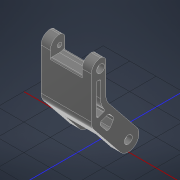
# Autodesk Inventor part: Swing-Arm B
Saved by Autodesk Inventor 2022.2 (Build 262287010, 287A)
## iProperties
Created: 2022-03-22
Part Number: Swing-Arm B
Material: ABS-Kunststoff
Document SubType Name: Modeling
Designer: sleib
Density: 1.06 g/cm^3
Appearance: Glatt - Schwarz
Author: sleib
Autodesk Inventor part; units mm, degrees
ref_plane "YZ Plane" through (0, 0, 0) normal (1, 0, 0) x (0, 1, 0)
ref_plane "XZ Plane" through (0, 0, 0) normal (0, 1, 0) x (-1, 0, 0)
ref_plane "XY Plane" through (0, 0, 0) normal (0, 0, 1) x (1, 0, 0)
sketch "SwingArm B" plane through (0, 0, 0) normal (0, 0, 1) x (1, 0, 0)
  arc A0 (25.4839, 28) -> (19.2029, 25.7813) centre (25.4839, 18) ccw
  arc A1 (37.33, 17) -> (31.049, 14.7813) centre (37.33, 7) ccw
  circle A2 centre (0, 0) radius 8 construction
  arc A3 (-5.0248, 6.2251) -> (5.0248, -6.2251) centre (0, 0) ccw
  line L0 (31.049, 14.7813) -> (5.0248, -6.2251)
  line L1 (19.2029, 25.7813) -> (-5.0248, 6.2251)
  line L2 (57, 28) -> (25.4839, 28)
  line L3 (60, 17) -> (37.33, 17)
  circle A4 centre (57, 21) radius 7 construction
  arc A5 (64, 21) -> (57, 28) centre (57, 21) ccw
  arc A6 (60, 17) -> (64, 21) centre (60, 21) ccw
  circle A7 centre (0, 0) radius 1.7
  circle A8 centre (57, 21) radius 1.7
  line L4 (57, 21) -> (26.0163, 21) construction
  line L5 (26.0163, 21) -> (0, 0) construction
  line L6 (22.6557, 20.0016) -> (24.0687, 16.0016)
  line L7 (23.4391, 13.7792) -> (20.7308, 11.5931)
  line L8 (18.4256, 11.4466) -> (14.8137, 13.6716)
  line L9 (14.6065, 16.9307) -> (19.5137, 20.8917)
  arc A9 (22.6557, 20.0016) -> (19.5137, 20.8917) centre (20.7699, 19.3355) ccw
  arc A10 (23.4391, 13.7792) -> (24.0687, 16.0016) centre (22.1829, 15.3355) ccw
  arc A11 (18.4256, 11.4466) -> (20.7308, 11.5931) centre (19.4746, 13.1494) ccw
  arc A12 (14.6065, 16.9307) -> (14.8137, 13.6716) centre (15.8627, 15.3744) ccw
  line L10 (22.1532, 27.429) -> (27.6033, 12) construction
  line L11 (37.33, 21) -> (60, 21) construction
  arc A13 (60, 21) -> (57, 24) centre (57, 21) ccw construction
  line L12 (57, 24) -> (25.4839, 24) construction
  arc A14 (25.4839, 24) -> (21.7153, 22.6688) centre (25.4839, 18) ccw construction
  line L13 (21.7153, 22.6688) -> (-2.5124, 3.1125) construction
  arc A15 (-2.5124, 3.1125) -> (2.5124, -3.1125) centre (0, 0) ccw construction
  line L14 (2.5124, -3.1125) -> (28.5366, 17.8939) construction
  arc A16 (37.33, 21) -> (28.5366, 17.8939) centre (37.33, 7) ccw construction
  line L15 (49.9641, 21.75) -> (50.2223, 22.75)
  line L16 (27.3731, 18.6564) -> (25.9565, 22.6669)
  line L17 (48.9958, 21) -> (37.33, 21)
  line L18 (49.254, 24) -> (26.8994, 24)
  arc A17 (37.33, 21) -> (28.917, 18.1902) centre (37.33, 7) ccw
  arc A18 (27.3731, 18.6564) -> (28.917, 18.1902) centre (28.316, 18.9895) ccw
  arc A19 (26.8994, 24) -> (25.9565, 22.6669) centre (26.8994, 23) ccw
  arc A20 (50.2223, 22.75) -> (49.254, 24) centre (49.254, 23) ccw
  arc A21 (48.9958, 21) -> (49.9641, 21.75) centre (48.9958, 22) ccw
  line L19 (17.0601, 18.9112) -> (22.0849, 12.6862) construction
  line L20 (13.0503, 15.6745) -> (18.0751, 9.4494) construction
  dimension "d0" = 3.4
  dimension "d1" = 3.4
  dimension "d2" = 57
  dimension "d3" = 21
  dimension "d4" = 141.09
  dimension "d5" = 4
  dimension "d6" = 7
  dimension "d7" = 4
  dimension "d10" = 10
  dimension "d11" = 10
  dimension "d13" = 2
  dimension "d14" = 2
  dimension "d42" = 16
  dimension "d43" = 4
  dimension "d45" = 1
  dimension "d46" = 4
  dimension "d49" = 20
  measures "d0" diameter of A7
  measures "d1" diameter of A8
  measures "d2" horizontal distance of L5.end L4.start
  measures "d3" vertical distance of L5.end L4.start
  measures "d4" angle of L5 L4
  measures "d5" distance from line of L3 L4.start
  measures "d6" distance from line of L4.start L2
  measures "d7" radius of A6
  measures "d10" radius of A1
  measures "d11" radius of A0
  measures "d13" radius of A9
  measures "d14" radius of A10
  measures "d42" diameter of A2
  measures "d43" distance between parallel lines of L3 L11
  measures "d45" radius of A20
  measures "d46" distance between parallel lines of L6 L16
  measures "d49" distance from line of point (0, 0) L20
sketch "Skizze1" plane through (0, 0, 0) normal (1, 0, 0) x (0, 1, 0)
  circle A0 centre (0, 0) radius 18
  arc A1 (52, 21) -> (54, 17) centre (57, 21) ccw
  line L0 (52, 21) -> (52, 28)
  arc A2 (25.4839, 28) -> (19.2029, 25.7813) centre (25.4839, 18) ccw
  arc A3 (37.33, 17) -> (31.049, 14.7813) centre (37.33, 7) ccw
  circle A4 centre (0, 0) radius 8 construction
  arc A5 (-5.0248, 6.2251) -> (5.0248, -6.2251) centre (0, 0) ccw
  line L1 (31.049, 14.7813) -> (5.0248, -6.2251)
  line L2 (19.2029, 25.7813) -> (-5.0248, 6.2251)
  line L3 (57, 28) -> (25.4839, 28)
  line L4 (60, 17) -> (37.33, 17)
  circle A6 centre (57, 21) radius 7 construction
  arc A7 (64, 21) -> (57, 28) centre (57, 21) ccw
  arc A8 (60, 17) -> (64, 21) centre (60, 21) ccw
  circle A9 centre (0, 0) radius 1.7
  circle A10 centre (57, 21) radius 1.7
  line L5 (57, 21) -> (26.0163, 21) construction
  line L6 (26.0163, 21) -> (0, 0) construction
  line L7 (22.6557, 20.0016) -> (24.0687, 16.0016)
  line L8 (23.4391, 13.7792) -> (20.7308, 11.5931)
  line L9 (18.4256, 11.4466) -> (14.8137, 13.6716)
  line L10 (14.6065, 16.9307) -> (19.5137, 20.8917)
  arc A11 (22.6557, 20.0016) -> (19.5137, 20.8917) centre (20.7699, 19.3355) ccw
  arc A12 (23.4391, 13.7792) -> (24.0687, 16.0016) centre (22.1829, 15.3355) ccw
  arc A13 (18.4256, 11.4466) -> (20.7308, 11.5931) centre (19.4746, 13.1494) ccw
  arc A14 (14.6065, 16.9307) -> (14.8137, 13.6716) centre (15.8627, 15.3744) ccw
  line L11 (22.1532, 27.429) -> (27.6033, 12) construction
  line L12 (37.33, 21) -> (60, 21) construction
  arc A15 (60, 21) -> (57, 24) centre (57, 21) ccw construction
  line L13 (57, 24) -> (25.4839, 24) construction
  arc A16 (25.4839, 24) -> (21.7153, 22.6688) centre (25.4839, 18) ccw construction
  line L14 (21.7153, 22.6688) -> (-2.5124, 3.1125) construction
  arc A17 (-2.5124, 3.1125) -> (2.5124, -3.1125) centre (0, 0) ccw construction
  line L15 (2.5124, -3.1125) -> (28.5366, 17.8939) construction
  arc A18 (37.33, 21) -> (28.5366, 17.8939) centre (37.33, 7) ccw construction
  line L16 (49.9641, 21.75) -> (50.2223, 22.75)
  line L17 (27.3731, 18.6564) -> (25.9565, 22.6669)
  line L18 (48.9958, 21) -> (37.33, 21)
  line L19 (49.254, 24) -> (26.8994, 24)
  arc A19 (37.33, 21) -> (28.917, 18.1902) centre (37.33, 7) ccw
  arc A20 (27.3731, 18.6564) -> (28.917, 18.1902) centre (28.316, 18.9895) ccw
  arc A21 (26.8994, 24) -> (25.9565, 22.6669) centre (26.8994, 23) ccw
  arc A22 (50.2223, 22.75) -> (49.254, 24) centre (49.254, 23) ccw
  arc A23 (48.9958, 21) -> (49.9641, 21.75) centre (48.9958, 22) ccw
  line L20 (17.0601, 18.9112) -> (22.0849, 12.6862) construction
  line L21 (13.0503, 15.6745) -> (18.0751, 9.4494) construction
  point P0 (17.5718, 3.9027)
  point P1 (7.5222, 16.3529)
  point P2 (-5.0248, 6.2251)
  point P3 (5.0248, -6.2251)
  point P4 (54, 17)
  dimension "d40" = 36
  dimension "d51" = 10
  constraints: 2 centre point, 2 end point, 2 point on circle, 1 tangent, 1 vertical, 6 other
  measures "d40" diameter of A0
  measures "d51" diameter of A1
extrude "Extrusion1" add sketch "Skizze1" along normal mid plane 38 contours L1 A5 L2 A0 | A0 L2 A2 L3 L0 A1 L4 A3 L1 | A1 L0 L3 A7 A8 L4 picked at (1.0334, 8.0558)
extrude "Extrusion6" cut sketch "Skizze1" along normal mid plane 24 contours L1 A5 L2 A0 | A1 L0 L3 A7 A8 L4 picked at (1.0334, 8.0558)
sketch "Skizze4" plane through (19, 0, 0) normal (1, 0, 0) x (0, 0, -1)
  circle A0 centre (0, 0) radius 3
  circle A1 centre (-21, 57) radius 1.7 projected
  circle A2 centre (-21, 57) radius 3
  dimension "d27" = 6
  dimension "d33" = 6
  constraints: 2 centre point, 2 coincident
  measures "d27" diameter of A0
  measures "d33" diameter of A2
extrude "Extrusion4" cut sketch "Skizze4" against normal blind 4
sketch "Skizze5" plane through (-19, 0, 0) normal (-1, 0, 0) x (0, 0, 1)
  line L0 (2.85, 1.6454) -> (2.85, -1.6454)
  line L1 (2.85, -1.6454) -> (0, -3.2909)
  line L2 (0, -3.2909) -> (-2.85, -1.6454)
  line L3 (-2.85, -1.6454) -> (-2.85, 1.6454)
  line L4 (-2.85, 1.6454) -> (0, 3.2909)
  line L5 (0, 3.2909) -> (2.85, 1.6454)
  circle A0 centre (21, 57) radius 1.7 projected
  line L6 (23.85, 58.6454) -> (23.85, 55.3546)
  line L7 (23.85, 55.3546) -> (21, 53.7091)
  line L8 (21, 53.7091) -> (18.15, 55.3546)
  line L9 (18.15, 55.3546) -> (18.15, 58.6454)
  line L10 (18.15, 58.6454) -> (21, 60.2909)
  line L11 (21, 60.2909) -> (23.85, 58.6454)
  line L12 (17, 60) -> (17, 37.33) projected
  point P0 (0, 0)
  point P1 (0, 0)
  dimension "d30" = 5.7
  dimension "d34" = 5.7
  constraints: 24 end point, 2 coincident, 2 parallel, 26 other
  measures "d30" distance between parallel lines of L2 L5
  measures "d34" distance between parallel lines of L6 L9
extrude "Extrusion5" cut sketch "Skizze5" against normal blind 4
fillet "Rundung1" radius 1 4 edges at (0, 54, 17) (0, 52, 28) (0, 17.5718, 3.9027) (0, 7.5222, 16.3529)
equation "\"d27\" = d33"
equation "\"d30\" = d34"
